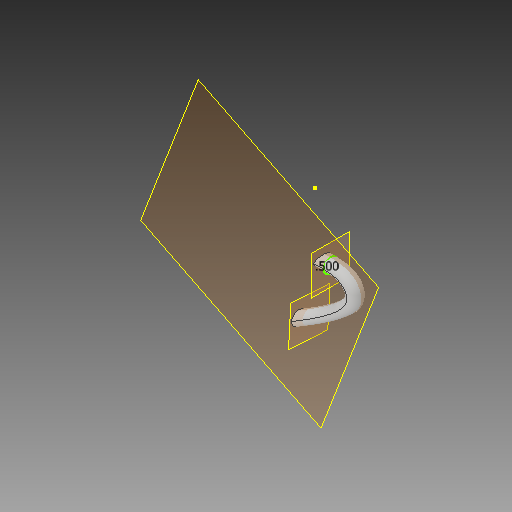
# Autodesk Inventor part: wire4
Saved by Autodesk Inventor 2018 (Build 220112000, 112)
## iProperties
Created: 2018-06-12
Part Number: wire4
Material: Generic
Document SubType Name: Modeling
Designer: DPLXuser
Density: 1 g/cm^3
Appearance: Default
Author: DPLXuser
Autodesk Inventor part; units mm, degrees
ref_plane "YZ Plane" through (0, 0, 0) normal (1, 0, 0) x (0, 1, 0)
ref_plane "XZ Plane" through (0, 0, 0) normal (0, 1, 0) x (-1, 0, 0)
ref_plane "XY Plane" through (0, 0, 0) normal (0, 0, 1) x (1, 0, 0)
ref_plane "Work Plane1" through (73.6831, -121.5246, -19.5504) normal (-0.0654948, -0.0766644, 0.9949035) x (0.4068709, 0.9083446, 0.0967789)
sketch "Sketch1" plane through (73.6831, -121.5246, -19.5504) normal (-0.0654948, -0.0766644, 0.9949035) x (0.4068709, 0.9083446, 0.0967789)
  spline S0 degree 2 poles (-2.253, 7.8234) (84.5394, -47.9586) (50.6543, 5.3958) knots 0 0 0 1 1 1
  point P0 (82.2988, 116.5451)
  point P1 (58.86, -19.5089)
  constraints: 3 other
ref_plane "Work Plane2" through (76.1191, -121.5284, -19.5011) normal (1, 0, 0) x (0, 0.0563932, 0.9984086)
sketch "Sketch2" plane through (76.1191, -121.5284, -19.5011) normal (1, 0, 0) x (0, 0.0563932, 0.9984086)
  circle A0 centre (0, 0) radius 6.35
  point P0 (26.3235, -120.2353)
  dimension "d0" = 12.7
  constraints: 1 centre point
  measures "d0" diameter of A0
ref_plane "Work Plane3" through (100.8932, -66.2199, -13.6083) normal (1, 0, 0) x (0, 0, 1)
sketch "Sketch3" plane through (100.8932, -66.2199, -13.6083) normal (1, 0, 0) x (0, 0, 1)
  circle A0 centre (0, 0) radius 6.35
  point P0 (13.6083, -66.2199)
  dimension "d1" = 12.7
  constraints: 1 centre point
  measures "d1" diameter of A0
sweep "Sweep1" add profiles "Sketch2" path "Sketch1"
body "Solid1"
